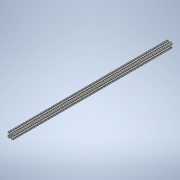
# Autodesk Inventor part: 30in 1x1 T slot
Saved by Autodesk Inventor 2020 (Build 240168000, 168)
## iProperties
Created: 2020-01-07
Part Number: 30in 1x1 T slot
Material: Generic
Document SubType Name: Modeling
Designer: 393735
Density: 1 g/cm^3
Appearance: Default
Author: 393735
Autodesk Inventor part; units mm, degrees
ref_plane "YZ Plane" through (0, 0, 0) normal (1, 0, 0) x (0, 1, 0)
ref_plane "XZ Plane" through (0, 0, 0) normal (0, 1, 0) x (-1, 0, 0)
ref_plane "XY Plane" through (0, 0, 0) normal (0, 0, 1) x (1, 0, 0)
sketch "Sketch1" plane through (0, 0, 0) normal (0, 0, 1) x (1, 0, 0)
  arc A0 (-5.4704, -4.1494) -> (-4.7072, -5.9944) centre (-4.7072, -4.914) ccw
  line L0 (-5.4704, -4.1494) -> (-2.243, -0.9279)
  arc A1 (0, 0) -> (-2.243, -0.9279) centre (0, -3.175) ccw
  line L1 (0, 0) -> (3.4185, 0)
  arc A2 (5.6615, -0.9279) -> (3.4185, 0) centre (3.4185, -3.175) ccw
  line L2 (5.6615, -0.9279) -> (8.8889, -4.1494)
  arc A3 (8.1257, -5.9944) -> (8.8889, -4.1494) centre (8.1257, -4.914) ccw
  line L3 (8.1257, -5.9944) -> (5.9968, -5.9944)
  arc A4 (5.9968, -5.9944) -> (4.9478, -7.0434) centre (5.9968, -7.0434) ccw
  line L4 (4.9478, -7.0434) -> (4.9478, -7.1552)
  arc A5 (4.9478, -7.1552) -> (5.9968, -8.2042) centre (5.9968, -7.1552) ccw
  line L5 (5.9968, -8.2042) -> (7.0264, -8.2042)
  arc A6 (8.0424, -8.2042) -> (7.0264, -8.2042) centre (7.5344, -8.2042) ccw
  line L6 (8.0424, -8.2042) -> (11.2597, -8.2042)
  arc A7 (12.2757, -8.204) -> (11.2597, -8.2042) centre (11.7677, -8.2042) ccw
  arc A8 (12.2757, -8.204) -> (14.4091, -6.0706) centre (12.3011, -6.096) ccw
  arc A9 (14.4093, -5.0546) -> (14.4091, -6.0706) centre (14.4093, -5.5626) ccw
  line L7 (14.4093, -5.0546) -> (14.4093, -1.8373)
  arc A10 (14.4093, -0.8213) -> (14.4093, -1.8373) centre (14.4093, -1.3293) ccw
  line L8 (14.4093, -0.8213) -> (14.4093, 0.2083)
  arc A11 (14.4093, 0.2083) -> (13.3602, 1.2573) centre (13.3602, 0.2083) ccw
  line L9 (13.3602, 1.2573) -> (13.2485, 1.2573)
  arc A12 (13.2485, 1.2573) -> (12.1995, 0.2083) centre (13.2485, 0.2083) ccw
  line L10 (12.1995, 0.2083) -> (12.1995, -1.9063)
  arc A13 (10.4464, -2.6336) -> (12.1995, -1.9063) centre (11.172, -1.9063) ccw
  line L11 (10.4464, -2.6336) -> (7.1503, 0.655)
  arc A14 (6.2178, 2.9026) -> (7.1503, 0.655) centre (9.3928, 2.9026) ccw
  line L12 (6.2178, 2.9026) -> (6.2178, 6.089)
  arc A15 (7.1503, 8.3366) -> (6.2178, 6.089) centre (9.3928, 6.089) ccw
  line L13 (7.1503, 8.3366) -> (10.4464, 11.6252)
  arc A16 (12.1995, 10.8979) -> (10.4464, 11.6252) centre (11.172, 10.8979) ccw
  line L14 (12.1995, 10.8979) -> (12.1995, 8.7833)
  arc A17 (12.1995, 8.7833) -> (13.2485, 7.7343) centre (13.2485, 8.7833) ccw
  line L15 (13.2485, 7.7343) -> (13.3602, 7.7343)
  arc A18 (13.3602, 7.7343) -> (14.4093, 8.7833) centre (13.3602, 8.7833) ccw
  line L16 (14.4093, 8.7833) -> (14.4093, 9.8129)
  arc A19 (14.4093, 10.8289) -> (14.4093, 9.8129) centre (14.4093, 10.3209) ccw
  line L17 (14.4093, 10.8289) -> (14.4093, 14.0462)
  arc A20 (14.4091, 15.0622) -> (14.4093, 14.0462) centre (14.4093, 14.5542) ccw
  arc A21 (14.4091, 15.0622) -> (12.2757, 17.1956) centre (12.3011, 15.0876) ccw
  arc A22 (11.2597, 17.1958) -> (12.2757, 17.1956) centre (11.7677, 17.1958) ccw
  line L18 (11.2597, 17.1958) -> (8.0424, 17.1958)
  arc A23 (7.0264, 17.1958) -> (8.0424, 17.1958) centre (7.5344, 17.1958) ccw
  line L19 (7.0264, 17.1958) -> (5.9968, 17.1958)
  arc A24 (5.9968, 17.1958) -> (4.9478, 16.1468) centre (5.9968, 16.1468) ccw
  line L20 (4.9478, 16.1468) -> (4.9478, 16.035)
  arc A25 (4.9478, 16.035) -> (5.9968, 14.986) centre (5.9968, 16.035) ccw
  line L21 (5.9968, 14.986) -> (8.186, 14.986)
  arc A26 (8.9163, 13.2202) -> (8.186, 14.986) centre (8.186, 13.9521) ccw
  line L22 (8.9163, 13.2202) -> (5.6075, 9.919)
  arc A27 (3.365, 8.9916) -> (5.6075, 9.919) centre (3.365, 12.1666) ccw
  line L23 (3.365, 8.9916) -> (0.0535, 8.9916)
  arc A28 (-2.189, 9.919) -> (0.0535, 8.9916) centre (0.0535, 12.1666) ccw
  line L24 (-2.189, 9.919) -> (-5.4978, 13.2202)
  arc A29 (-4.7675, 14.986) -> (-5.4978, 13.2202) centre (-4.7675, 13.9521) ccw
  line L25 (-4.7675, 14.986) -> (-2.5783, 14.986)
  arc A30 (-2.5783, 14.986) -> (-1.5292, 16.035) centre (-2.5783, 16.035) ccw
  line L26 (-1.5292, 16.035) -> (-1.5292, 16.1468)
  arc A31 (-1.5292, 16.1468) -> (-2.5783, 17.1958) centre (-2.5783, 16.1468) ccw
  line L27 (-2.5783, 17.1958) -> (-3.6079, 17.1958)
  arc A32 (-4.6239, 17.1958) -> (-3.6079, 17.1958) centre (-4.1159, 17.1958) ccw
  line L28 (-4.6239, 17.1958) -> (-7.8412, 17.1958)
  arc A33 (-8.8572, 17.1956) -> (-7.8412, 17.1958) centre (-8.3492, 17.1958) ccw
  arc A34 (-8.8572, 17.1956) -> (-10.9906, 15.0622) centre (-8.8825, 15.0876) ccw
  arc A35 (-10.9907, 14.0462) -> (-10.9906, 15.0622) centre (-10.9907, 14.5542) ccw
  line L29 (-10.9907, 14.0462) -> (-10.9907, 10.8289)
  arc A36 (-10.9907, 9.8129) -> (-10.9907, 10.8289) centre (-10.9907, 10.3209) ccw
  line L30 (-10.9907, 9.8129) -> (-10.9907, 8.7833)
  arc A37 (-10.9907, 8.7833) -> (-9.9417, 7.7343) centre (-9.9417, 8.7833) ccw
  line L31 (-9.9417, 7.7343) -> (-9.83, 7.7343)
  arc A38 (-9.83, 7.7343) -> (-8.7809, 8.7833) centre (-9.83, 8.7833) ccw
  line L32 (-8.7809, 8.7833) -> (-8.7809, 10.8979)
  arc A39 (-7.0279, 11.6252) -> (-8.7809, 10.8979) centre (-7.7535, 10.8979) ccw
  line L33 (-7.0279, 11.6252) -> (-3.7318, 8.3366)
  arc A40 (-2.7992, 6.089) -> (-3.7318, 8.3366) centre (-5.9742, 6.089) ccw
  line L34 (-2.7992, 6.089) -> (-2.7992, 2.9026)
  arc A41 (-3.7318, 0.655) -> (-2.7992, 2.9026) centre (-5.9742, 2.9026) ccw
  line L35 (-3.7318, 0.655) -> (-7.0279, -2.6336)
  arc A42 (-8.7809, -1.9063) -> (-7.0279, -2.6336) centre (-7.7535, -1.9063) ccw
  line L36 (-8.7809, -1.9063) -> (-8.7809, 0.2083)
  arc A43 (-8.7809, 0.2083) -> (-9.83, 1.2573) centre (-9.83, 0.2083) ccw
  line L37 (-9.83, 1.2573) -> (-9.9417, 1.2573)
  arc A44 (-9.9417, 1.2573) -> (-10.9907, 0.2083) centre (-9.9417, 0.2083) ccw
  line L38 (-10.9907, 0.2083) -> (-10.9907, -0.8213)
  arc A45 (-10.9907, -1.8373) -> (-10.9907, -0.8213) centre (-10.9907, -1.3293) ccw
  line L39 (-10.9907, -1.8373) -> (-10.9907, -5.0546)
  arc A46 (-10.9906, -6.0706) -> (-10.9907, -5.0546) centre (-10.9907, -5.5626) ccw
  arc A47 (-10.9906, -6.0706) -> (-8.8572, -8.204) centre (-8.8825, -6.096) ccw
  arc A48 (-7.8412, -8.2042) -> (-8.8572, -8.204) centre (-8.3492, -8.2042) ccw
  line L40 (-7.8412, -8.2042) -> (-4.6239, -8.2042)
  arc A49 (-3.6079, -8.2042) -> (-4.6239, -8.2042) centre (-4.1159, -8.2042) ccw
  line L41 (-3.6079, -8.2042) -> (-2.5783, -8.2042)
  arc A50 (-2.5783, -8.2042) -> (-1.5292, -7.1552) centre (-2.5783, -7.1552) ccw
  line L42 (-1.5292, -7.1552) -> (-1.5292, -7.0434)
  arc A51 (-1.5292, -7.0434) -> (-2.5783, -5.9944) centre (-2.5783, -7.0434) ccw
  line L43 (-2.5783, -5.9944) -> (-4.7072, -5.9944)
  circle A52 centre (1.7093, 4.4958) radius 2.6035
  constraints: 104 point on circle, 88 end point, 53 centre point
extrude "Extrusion1" add sketch "Sketch1" along normal blind 762
body "Solid1"
